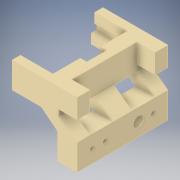
# Autodesk Inventor part: Body_lateralized
Saved by Autodesk Inventor 2020 (Build 240168000, 168)
## iProperties
Created: 2019-02-19
Part Number: Body_lateralized
Material: 일반
Document SubType Name: Modeling
Designer: Jeong Ji Hoon
Density: 1 g/cm^3
Appearance: 기본값
Author: Jeong Ji Hoon
## iProperties of the stored document _3D 인쇄.ipt
Created: 2019-12-02
Part Number: _3D 인쇄
Material: 일반
Document SubType Name: Modeling
Designer: Knowblesse
Density: 1 g/cm^3
Appearance: 기본값
Author: Knowblesse
Autodesk Inventor part; units mm, degrees
ref_plane "YZ Plane" through (0, 0, 0) normal (1, 0, 0) x (0, 1, 0)
ref_plane "XZ Plane" through (0, 0, 0) normal (0, 1, 0) x (-1, 0, 0)
ref_plane "XY Plane" through (0, 0, 0) normal (0, 0, 1) x (1, 0, 0)
sketch "스케치1" plane through (0, 0, 0) normal (0, 1, 0) x (-1, 0, 0)
  line L0 (0, 0) -> (0, -14)
  line L1 (0, -14) -> (7.2, -14)
  line L2 (0, 0) -> (7.2, 0)
  line L3 (7.2, 0) -> (7.2, -1.8)
  line L4 (7.2, -1.8) -> (2.7, -1.8)
  line L5 (2.7, -1.8) -> (2.7, -5.5)
  line L6 (2.7, -5.5) -> (1.2, -5.5)
  line L7 (1.2, -5.5) -> (1.2, -8.5)
  line L8 (1.2, -8.5) -> (2.7, -8.5)
  line L9 (2.7, -8.5) -> (2.7, -12.2)
  line L10 (2.7, -12.2) -> (7.2, -12.2)
  line L11 (7.2, -12.2) -> (7.2, -14)
  line L12 (7.2, -0.95) -> (1.2, -0.95) construction
  line L13 (1.2, -0.95) -> (1.2, -13.05) construction
  line L14 (1.2, -13.05) -> (7.2, -13.05) construction
  dimension "d0" = 14
  dimension "d2" = 7.2
  dimension "d3" = 1.8
  dimension "d5" = 3.7
  dimension "d6" = 1.5
  dimension "d7" = 3
  dimension "d8" = 1.5
  dimension "d9" = 3.7
  dimension "d47" = 12.1
  dimension "d48" = 0.85
  dimension "d49" = 0.85
  dimension "d63" = 6
  constraints: 30 end point, 5 horizontal, 5 vertical, 4 point on line, 3 perpendicular, 2 collinear
  measures "d0" distance of L0.start L0.end
  measures "d2" distance of L0.start L2.end
  measures "d3" distance of L2.end L3.end
  measures "d5" distance of L4.end L5.end
  measures "d6" distance of L5.end L6.end
  measures "d7" distance of L6.end L7.end
  measures "d8" distance of L7.end L8.end
  measures "d9" distance of L8.end L9.end
  measures "d47" distance between parallel lines of L14 L12
  measures "d48" distance between parallel lines of L12 L4
  measures "d49" distance between parallel lines of L10 L14
  measures "d63" distance between parallel lines of L13 L3
extrude "돌출1" add sketch "스케치1" along normal blind 4
sketch "스케치9" plane through (-7.2, 0, -14) normal (-1, 0, 0) x (0, 0, 1)
  line L0 (12.2, 0) -> (14, 0) projected
  line L1 (14, 0) -> (14, 4) projected
  line L2 (12.2, 4) -> (14, 4) projected
  line L3 (12.2, 0) -> (12.2, 4) projected
  line L4 (0, 0) -> (1.8, 0) projected
  line L5 (1.8, 0) -> (1.8, 4) projected
  line L6 (0, 4) -> (1.8, 4) projected
  line L7 (0, 0) -> (0, 4) projected
  line L8 (13.05, 1.5) -> (0.95, 1.5)
  line L9 (0.95, 1.5) -> (0.95, 2.5)
  line L10 (0.95, 2.5) -> (13.05, 2.5)
  line L11 (13.05, 2.5) -> (13.05, 1.5)
  dimension "d55" = 0.95
  dimension "d56" = 0.95
  dimension "d60" = 1
  dimension "d61" = 1.5
  dimension "d62" = 1.5
  dimension "d71" = 12.1
  constraints: 8 end point, 2 parallel, 1 horizontal, 1 perpendicular
  measures "d55" distance between parallel lines of L1 L11
  measures "d56" distance between parallel lines of L7 L9
  measures "d60" distance of L10.end L8.start
  measures "d61" distance between parallel lines of L0 L8
  measures "d62" distance between parallel lines of L2 L10
  measures "d71" distance of L9.end L10.end
extrude "돌출9" cut sketch "스케치9" against normal blind 6 contours L8 L5 L10 L3 | L3 L10 L11 L8 | L8 L9 L10 L5
sketch "스케치12" plane through (0, 0, -14) normal (0, 0, -1) x (-1, 0, 0)
  line L0 (0, 0) -> (7.2, 0) projected
  line L1 (7.2, 0) -> (7.2, 4) projected
  line L2 (0, 4) -> (7.2, 4) projected
  line L3 (0, 0) -> (0, 4) projected
  line L4 (0.2, -2) -> (-2.8, -2)
  line L5 (-2.8, -2) -> (-2.8, -6)
  line L6 (-2.8, -6) -> (0.2, -6)
  line L7 (0.2, -6) -> (0.2, -2)
  line L8 (2.7, 1.5) -> (1.2, 1.5) projected
  line L9 (1.2, 0) -> (1.2, 1.5) projected
  line L10 (1.2, 0) -> (2.7, 0) projected
  line L11 (2.7, 0) -> (2.7, 1.5) projected
  line L12 (0, 0) -> (0, 4) projected
  line L13 (0, 0) -> (-2.8, -2)
  line L14 (2.7, 0) -> (2.7, 1.5) projected
  line L15 (2.7, 0) -> (0.2, -2)
  dimension "d72" = 3
  dimension "d73" = 4
  dimension "d76" = 2
  dimension "d77" = 10
  constraints: 12 end point, 2 parallel, 1 horizontal, 1 perpendicular
  measures "d72" distance of L6.end L5.end
  measures "d73" distance of L4.end L5.end
  measures "d76" distance between parallel lines of L0 L4
  measures "d77" distance between parallel lines of L5 L1
extrude "돌출12" add sketch "스케치12" against normal up to surface (14 mm away) contours L0 L15 L4 L13 | L4 L7 L6 L5
sketch "스케치14" plane through (-2.7, 1.5, -12.2) normal (-1, 0, 0) x (0, 0, 1)
  line L0 (12.2, -1.5) -> (-1.8, -1.5) projected
  line L1 (-1.8, -3.5) -> (12.2, -3.5) projected
  line L2 (-1.8, -1.5) -> (0.2, -1.5)
  line L3 (0.2, -1.5) -> (0.2, -3.5)
  line L4 (0.2, -3.5) -> (-1.8, -3.5)
  line L5 (-1.8, -3.5) -> (-1.8, -1.5)
  line L6 (12.2, -1.5) -> (10.2, -1.5)
  line L7 (10.2, -1.5) -> (10.2, -3.5)
  line L8 (10.2, -3.5) -> (12.2, -3.5)
  line L9 (12.2, -3.5) -> (12.2, -1.5)
  line L10 (3.7, -1.5) -> (6.7, -1.5)
  line L11 (6.7, -1.5) -> (6.7, -3.5)
  line L12 (6.7, -3.5) -> (3.7, -3.5)
  line L13 (3.7, -3.5) -> (3.7, -1.5)
  line L14 (3.7, -1.5) -> (3.7, 0) projected
  point P0 (6.7, -1.5)
  point P1 (10.2, -3.5)
  point P2 (3.7, -1.5)
  point P3 (0.2, -1.5)
  dimension "d86" = 2
  dimension "d87" = 2
  dimension "d88" = 3
  constraints: 24 end point, 6 parallel, 5 point on line, 3 horizontal, 3 perpendicular
  measures "d86" distance of L3.end L4.end
  measures "d87" distance of L8.end L7.end
  measures "d88" distance of L11.end L12.end
extrude "돌출13" cut sketch "스케치14" against normal up to surface (5.5 mm away) contours L7 L1 L11 L0 | L13 L1 L3 L0
sketch "스케치15" plane through (-0.2, -6, -14) normal (-1, 0, 0) x (0, 0, 1)
  line L0 (14, 0) -> (14, 4) construction
  line L1 (14, 2) -> (0, 2) construction
  line L2 (0, 0) -> (0, 4) construction
  point P0 (14, 6)
  point P1 (11.7, 2)
  point P2 (9.7, 2)
  point P3 (4.5, 2)
  point P4 (2.3, 2)
  dimension "d91" = 2.3
  dimension "d92" = 2.3
  dimension "d95" = 2.2
  dimension "d96" = 5.2
  dimension "d128" = 2
  constraints: 4 point on line, 2 end point, 2 midpoint
  measures "d91" distance from line of point (2.3, 2) L2
  measures "d92" distance from line of L0 point (11.7, 2)
  measures "d95" distance of point (4.5, 2) point (2.3, 2)
  measures "d96" distance of point (9.7, 2) point (4.5, 2)
  measures "d128" distance of point (11.7, 2) point (9.7, 2)
hole "구멍1" at (-0.2, -4, -4.3) direction (1, 0, 0) diameter 0.65 end through all
hole "구멍2" at (-0.2, -4, -9.5) direction (1, 0, 0) diameter 1.6 end through all
hole "구멍3" at (-0.2, -4, -2.3) at (-0.2, -4, -11.7) direction (1, 0, 0) diameter 0.63 end through all
sketch "스케치17" plane through (0, 4, 0) normal (0, 1, 0) x (1, 0, 0)
  line L0 (0, 0) -> (0, 14) projected
  line L1 (0, 14) -> (-7.2, 14) projected
  line L2 (-7.2, 14) -> (-7.2, 12.2) projected
  line L3 (-7.2, 12.2) -> (-2.7, 12.2) projected
  line L4 (-2.7, 12.2) -> (-2.7, 8.5) projected
  line L5 (-2.7, 8.5) -> (-1.2, 8.5) projected
  line L6 (-1.2, 8.5) -> (-1.2, 5.5) projected
  line L7 (-1.2, 5.5) -> (-2.7, 5.5) projected
  line L8 (-2.7, 5.5) -> (-2.7, 1.8) projected
  line L9 (-2.7, 1.8) -> (-7.2, 1.8) projected
  line L10 (-7.2, 1.8) -> (-7.2, 0) projected
  line L11 (-7.2, 0) -> (0, 0) projected
  line L12 (-7.2, 1.8) -> (-7.2, 0) projected
  line L13 (-7.2, 1.3) -> (-2.2, 1.3)
  line L14 (-2.2, 1.3) -> (-2.2, 12.7)
  line L15 (-2.2, 12.7) -> (-7.2, 12.7)
  line L16 (-7.2, 12.7) -> (-7.2, 1.3)
  point P0 (-7.2, 12.7)
  dimension "d118" = 0.5
  dimension "d119" = 0.5
  dimension "d120" = 0.5
  constraints: 8 end point, 2 parallel, 1 horizontal, 1 perpendicular, 1 point on line
  measures "d118" distance between parallel lines of L13 L9
  measures "d119" distance between parallel lines of L15 L3
  measures "d120" distance between parallel lines of L4 L14
extrude "돌출14" cut sketch "스케치17" against normal up to surface (1.5 mm away) contours L10 L9 L8 L7 L14 L13 | L15 L14 L5 L4 L3 L2 | L16 L3 L4 L5 L14 L7 L8 L9
sketch "스케치18" plane through (0, 4, 0) normal (1, 0, 0) x (0, 0, -1)
  line L0 (0, 0) -> (14, 0) projected
  line L1 (14, -6) -> (12, -6) projected
  line L2 (14, 0) -> (12, 0)
  line L3 (12, 0) -> (12, -6)
  line L4 (12, -6) -> (14, -6)
  line L5 (14, -6) -> (14, 0)
  line L6 (0, -4) -> (0, 0) projected
  line L7 (2, -4) -> (2, -6) projected
  line L8 (0, 0) -> (2, 0)
  line L9 (2, 0) -> (2, -6)
  line L10 (2, -6) -> (0, -6)
  line L11 (0, -6) -> (0, 0)
  constraints: 16 end point, 4 parallel, 2 horizontal, 2 perpendicular
extrude "돌출15" add sketch "스케치18" along normal up to surface (2.8 mm away)
sketch "스케치20" plane through (-7.2, 0, -14) normal (0, 0, -1) x (-1, 0, 0)
  line L0 (-10, -2) -> (-10, 4) projected
  line L1 (-10, 1) -> (-10, -2)
  line L2 (-7.2, 0) -> (-7.2, 4) projected
  line L3 (-10, -2) -> (-7.2, 0)
  line L4 (-7.2, 0) -> (-10, -2) projected
  line L5 (-7.2, 0) -> (-7.2, 1)
  line L6 (-10, 1) -> (-7.2, 1)
  constraints: 8 end point, 1 collinear, 1 midpoint, 1 perpendicular, 1 point on line
extrude "돌출16" cut sketch "스케치20" against normal through all
equation "\"d5\" = d9"
equation "\"d9\" = 0.5 * d0 - 0.5 * d7 - d3"
equation "\"d48\" = d49"
equation "\"d55\" = d56"
equation "\"d61\" = d62"
